HousingBase_v15 (Autodesk Fusion 360 design; units mm, degrees)
Autodesk Fusion 360 part; units mm, degrees
note: some values were not read from the file. Set by a fixed rule: the direction of a hole.
sketch "Sketch1" plane through (0, 0, 0) normal (0, 0, 1) x (1, 0, 0)
  circle A0 centre (0, 0) radius 19.05
  circle A1 centre (0, 0) radius 25.4
  circle A2 centre (0, 0) radius 22.225 construction
  line L0 (0, 0) -> (0, 11.0018) construction
  circle A3 centre (0, 0) radius 7.9375 construction
  circle A4 centre (0, 11.0018) radius 1.8415
  line L1 (-16.9425, 18.9238) -> (16.9425, 18.9238) construction
  line L2 (2.1891, 18.9238) -> (1.8397, 10.9214)
  line L3 (-2.1891, 18.9238) -> (-1.8397, 10.9214)
  circle A5 centre (0, 11.0018) radius 3.0643 construction
  point P0 (0, 18.9238)
  point P1 (0, 22.225)
  dimension "d1" = 38.1
  dimension "d2" = 50.8
  dimension "d3" = 44.45
  dimension "d4" = 11.0018
  dimension "d5" = 15.875
  dimension "otherdiam" = 3.683
  dimension "d28" = 2.5
  constraint coincident A0.centre A1.centre
  constraint concentric A1 A2
  constraint concentric A0 A3
  constraint coincident L0.end A4.centre
  constraint horizontal L1
  constraint midpoint P0 L1
  constraint coincident A1 L1.end
  constraint vertical L0
  constraint vertical A0.centre P0
  constraint coincident L1 L2.start
  constraint tangent A4 L2
  constraint coincident A4 L2.end
  constraint symmetric L0 L2.start L3.start
  constraint symmetric L0 L2.end L3.end
  constraint coincident A0 L2.start
  constraint coincident A2 P1
  constraint vertical A0.centre P1
  constraint tangent A3 A5
  constraint concentric A4 A5
  measures "d1" diameter of A0
  measures "d2" diameter of A1
  measures "d3" diameter of A2
  measures "d4" distance of A0.centre L0.end
  measures "d5" diameter of A3
  measures "otherdiam" diameter of A4
  measures "d28" angle of L0 L2
extrude "Extrude1" add sketch "Sketch1" along normal blind 12.7
extrude "Extrude2" add sketch "Sketch1" along normal blind 3.175 contours A0 A4 L2 L3 | A4 L2 picked at (-0.0134, 16.9716)
hole "Hole1" at (0, 22.225, 0) direction (0, 0, 1) diameter 4.4958 end up to surface (12.7 mm away)
hole "Hole2" at (0, 11.0018, 0) direction (0, 0, 1) diameter 2.4384 end up to surface (3.175 mm away)
pattern_circular "C-Pattern1" count 3 over 360 about axis through (0, 0, 0) along (0, 0, 1) of "Extrude2"
pattern_circular "C-Pattern2" count 3 over 360 about axis through (0, 0, 0) along (0, 0, 1) of "Hole1"
pattern_circular "C-Pattern3" count 3 over 360 about axis through (0, 0, 0) along (0, 0, 1) of "Hole2"
fillet "Fillet1" radius 4.7625 6 edges at (-17.4831, -7.5661, 1.5875) (-15.2939, -11.3577, 1.5875) (2.1891, 18.9238, 1.5875) (-2.1891, 18.9238, 1.5875) (15.2939, -11.3577, 1.5875) (17.4831, -7.5661, 1.5875)
equation "d28 = angle"
equation "angle = 2.5 deg"
